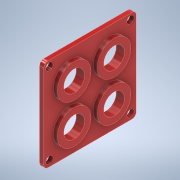
# Autodesk Inventor part: BatteryRoof
Saved by Autodesk Inventor 2022 (Build 260153000, 153)
## iProperties
Created: 2022-04-11
Part Number: BatteryRoof
Material: ABS Plastic
Document SubType Name: Modeling
Designer: ForseFire
Density: 1.06 g/cm^3
Appearance: Red
Author: ForseFire
Autodesk Inventor part; units mm, degrees
ref_plane "YZ Plane" through (0, 0, 0) normal (1, 0, 0) x (0, 1, 0)
ref_plane "XZ Plane" through (0, 0, 0) normal (0, 1, 0) x (-1, 0, 0)
ref_plane "XY Plane" through (0, 0, 0) normal (0, 0, 1) x (1, 0, 0)
sketch "Sketch1" plane through (0, 0, 0) normal (1, 0, 0) x (0, 1, 0)
  line L0 (-22, -22) -> (22, -22)
  line L1 (22, -22) -> (22, 22)
  line L2 (22, 22) -> (-22, 22)
  line L3 (-22, 22) -> (-22, -22)
  line L4 (-22, -22) -> (22, 22) construction
  line L5 (22, -22) -> (-22, 22) construction
  line L6 (-19.3, -19.3) -> (19.3, -19.3)
  line L7 (19.3, -19.3) -> (19.3, 19.3)
  line L8 (19.3, 19.3) -> (-19.3, 19.3)
  line L9 (-19.3, 19.3) -> (-19.3, -19.3)
  line L10 (-19.3, -19.3) -> (19.3, 19.3) construction
  line L11 (19.3, -19.3) -> (-19.3, 19.3) construction
  circle A0 centre (19.3, 19.3) radius 1.75
  circle A1 centre (19.3, -19.3) radius 1.75
  circle A2 centre (-19.3, -19.3) radius 1.75
  circle A3 centre (-19.3, 19.3) radius 1.75
  line L12 (19.3, 0) -> (0, 0)
  circle A4 centre (9.5, -9.5) radius 5
  circle A5 centre (9.5, 9.5) radius 5
  line L13 (0, 0) -> (-19.3, 0)
  circle A6 centre (-9.5, -9.5) radius 5
  circle A7 centre (-9.5, 9.5) radius 5
  circle A8 centre (9.5, -9.5) radius 9.5
  circle A9 centre (9.5, 9.5) radius 9.5
  circle A10 centre (-9.5, 9.5) radius 9.5
  circle A11 centre (-9.5, -9.5) radius 9.5
  point P0 (0, 0)
  point P1 (0, 0)
  point P2 (6.364, 6.364)
  dimension "d0" = 44
  dimension "d1" = 44
  dimension "d6" = 38.6
  dimension "d7" = 38.6
  dimension "d8" = 3.5
  dimension "d9" = 3.5
  dimension "d10" = 3.5
  dimension "d11" = 3.5
  dimension "d19" = 10
  dimension "d20" = 10
  dimension "d21" = 10
  dimension "d22" = 10
  dimension "d23" = 19
  dimension "d24" = 19
  dimension "d25" = 19
  dimension "d26" = 19
  constraints: 28 end point, 12 centre point, 8 coincident, 8 midpoint, 5 point on line, 4 parallel, 3 equal radius, 2 horizontal, 2 perpendicular, 1 vertical alignment
  measures "d0" distance of L2.end L1.end
  measures "d1" distance of L0.end L1.end
  measures "d6" distance of L8.end L7.end
  measures "d7" distance of L6.end L7.end
  measures "d8" diameter of A0
  measures "d9" diameter of A1
  measures "d10" diameter of A2
  measures "d11" diameter of A3
  measures "d19" diameter of A4
  measures "d20" diameter of A5
  measures "d21" diameter of A6
  measures "d22" diameter of A7
  measures "d23" diameter of A8
  measures "d24" diameter of A9
  measures "d25" diameter of A10
  measures "d26" diameter of A11
extrude "Extrusion1" add sketch "Sketch1" along normal blind 2 contours L3 L2 L1 L0 | A2 L9 L13 A11 A8 L12 L7 A1 L6 | L9 A3 L8 A0 L7 L12 A9 A10 L13 | A10 A9 L12 L13 | A10 | L13 L12 A8 A11 | A11 | A9 | A8
fillet "Fillet1" radius 2 4 edges at (1, -22, 22) (1, -22, -22) (1, 22, -22) (1, 22, 22)
sketch "Sketch2" plane through (2, 0, 0) normal (1, 0, 0) x (0, 0, -1)
  arc A0 (-20, 22) -> (-22, 20) centre (-20, 20) ccw projected
  line L0 (-22, 20) -> (-22, -20) projected
  arc A1 (-22, -20) -> (-20, -22) centre (-20, -20) ccw projected
  line L1 (-20, -22) -> (20, -22) projected
  arc A2 (20, -22) -> (22, -20) centre (20, -20) ccw projected
  line L2 (22, -20) -> (22, 20) projected
  arc A3 (22, 20) -> (20, 22) centre (20, 20) ccw projected
  line L3 (20, 22) -> (-20, 22) projected
  circle A4 centre (-19.3, -19.3) radius 1.75 projected
  circle A5 centre (19.3, -19.3) radius 1.75 projected
  circle A6 centre (9.5, 9.5) radius 5 projected
  circle A7 centre (9.5, -9.5) radius 5 projected
  circle A8 centre (19.3, 19.3) radius 1.75 projected
  circle A9 centre (-9.5, 9.5) radius 5 projected
  circle A10 centre (-9.5, -9.5) radius 5 projected
  circle A11 centre (-19.3, 19.3) radius 1.75 projected
  circle A12 centre (-9.5, -9.5) radius 8
  circle A13 centre (-9.5, 9.5) radius 8
  circle A14 centre (9.5, 9.5) radius 8
  circle A15 centre (9.5, -9.5) radius 8
  point P0 (0, 0)
  dimension "d27" = 16
  dimension "d28" = 16
  dimension "d29" = 16
  dimension "d30" = 16
  constraints: 4 centre point, 4 coincident
  measures "d27" diameter of A12
  measures "d28" diameter of A13
  measures "d29" diameter of A14
  measures "d30" diameter of A15
extrude "Extrusion2" add sketch "Sketch2" along normal blind 2 contours A12 | A13 | A14 | A15
body "Solid1"
